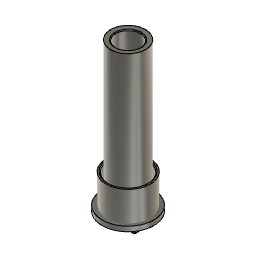
Tripod-mount v6 (Autodesk Fusion 360 design; units mm, degrees)
Autodesk Fusion 360 part; units mm, degrees
cylinder "CylinderPrimitive1" add diameter 53 height 5 placed x (1, 0, 0) y (0, 1, 0) z (0, 0, 1) at (0, 0, 0) makes body 1
hole "Hole1" at (0, 0.0929, 5) direction (0, 0, -1) diameter 40.2 depth 3 tip angle 180 countersink diameter 40.3 countersink angle 90 bodies 1
cylinder "CylinderPrimitive2" add diameter 35.8 height 150 placed x (1, 0, 0) y (0, 1, 0) z (0, 0, 1) at (0, 0.0929, 2) bodies 1
hole "Hole2" at (0.2787, -0.1858, 152) direction (0, 0, -1) diameter 25.5 depth 200 tip angle 180 countersink diameter 27 countersink angle 90 bodies 1
cylinder "CylinderPrimitive3" add diameter 2.9 height 5 placed x (1, 0, 0) y (0, 1, 0) z (0, 0, 1) at (20, -30, 0) separate body makes body 2
move_body "Move1" bodies 2 to x (1, 0, 0) y (0, 1, 0) z (0, 0, 1) at (3.3607, -17.8119, 0)
move_body "Move2" bodies 2 to x (1, 0, 0) y (0, 1, 0) z (0, 0, 1) at (-13.1273, 4.733, 0)
pattern_circular "C-Pattern1" count 3 over 360 about axis through (0, 0, 1.75) along (0, 0, 1) of bodies 2 makes body 3 at (31.404, 31.6199, 3.3333) makes body 4 at (-42.6759, 11.2491, 1.6667)
move_body "MoveFace1" bodies 3 to x (1, 0, 0) y (0, 1, 0) z (0, 0, 1) at (-14.7703, -15.636, -10.1255) on bodies 3
sketch "Sketch4" plane through (0, 0, 0) normal (1, 0, 0) x (0, 1, 0)
move_body "Move6" bodies 3 to x (1, 0, 0) y (0, 1, 0) z (0, 0, 1) at (0.1863, -0.8041, 5.3323)
move_body "Move7" bodies 3 to x (1, 0, 0) y (0, 1, 0) z (0, 0, 1) at (-17.5558, 9.3545, 0)
move_body "Move8" bodies 4 to x (1, 0, 0) y (0, 1, 0) z (0, 0, 1) at (22.6561, -23.0272, -5.0478)
move_body "Move10" bodies 2 to x (1, 0, 0) y (0, 1, 0) z (0, 0, 1) at (-7.5029, 18.5186, -9.6276)
move_body "Move11" bodies 2 to x (1, 0, 0) y (0, 1, 0) z (0, 0, 1) at (15.121, 9.8671, 0)
move_body "Move12" bodies 3 to x (1, 0, 0) y (0, 1, 0) z (0, 0, 1) at (-0.897, -0.7689, 0)
move_body "Move13" bodies 2 to x (1, 0, 0) y (0, 1, 0) z (0, 0, 1) at (-0.6407, 1.9222, 4.8344)
move_body "Move14" bodies 3 to x (1, 0, 0) y (0, 1, 0) z (0, 0, 1) at (1.0252, -0.2563, 0)
move_body "Move15" bodies 4 to x (1, 0, 0) y (0, 1, 0) z (0, 0, 1) at (0.7689, -0.5126, 0)
move_body "Move16" bodies 3 to x (1, 0, 0) y (0, 1, 0) z (0, 0, 1) at (-0.2563, -0.2563, 0)
move_body "Move17" bodies 3 to x (1, 0, 0) y (0, 1, 0) z (0, 0, 1) at (0.1281, -0.6407, 0)
move_body "Move18" bodies 4 to x (1, 0, 0) y (0, 1, 0) z (0, 0, 1) at (0.3844, 0.3844, 0)
move_body "Move19" bodies 2 to x (1, 0, 0) y (0, 1, 0) z (0, 0, 1) at (-0.5126, 0.5126, 0)
move_body "Move20" bodies 3 to x (1, 0, 0) y (0, 1, 0) z (0, 0, 1) at (0, -0.5126, 0)
move_body "Move21" bodies 4 to x (1, 0, 0) y (0, 1, 0) z (0, 0, 1) at (0.5126, 0.5126, 0)
move_body "Move22" bodies 2 to x (1, 0, 0) y (0, 1, 0) z (0, 0, 1) at (0.3844, 0.5126, 0)
move_body "Move23" bodies 2 to x (1, 0, 0) y (0, 1, 0) z (0, 0, 1) at (0.6407, 0.7689, 0)
move_body "Move24" bodies 4 to x (1, 0, 0) y (0, 1, 0) z (0, 0, 1) at (-0.7689, 0.1281, 0)
move_body "Move25" bodies 4 to x (1, 0, 0) y (0, 1, 0) z (0, 0, 1) at (0.2563, 0.2563, 0)
move_body "Move26" bodies 2 to x (1, 0, 0) y (0, 1, 0) z (0, 0, 1) at (-0.1281, -0.1281, 0)
move_body "Move27" bodies 4 to x (1, 0, 0) y (0, 1, 0) z (0, 0, 1) at (0.3844, 0, 0)
move_body "Move28" bodies 4 to x (1, 0, 0) y (0, 1, 0) z (0, 0, 1) at (-0.3844, 0, 0)
move_body "Move29" bodies 4 to x (1, 0, 0) y (0, 1, 0) z (0, 0, 1) at (0.2563, -0.1281, 0)
move_body "Move30" bodies 3 to x (1, 0, 0) y (0, 1, 0) z (0, 0, 1) at (0.3844, -0.2563, 0)
move_body "Move31" bodies 3 to x (1, 0, 0) y (0, 1, 0) z (0, 0, 1) at (0.2563, 0.2563, 0)
move_body "Move32" bodies 3 to x (1, 0, 0) y (0, 1, 0) z (0, 0, 1) at (0, -0.1281, 0)
cylinder "CylinderPrimitive4" add diameter 45 height 35 placed x (1, 0, 0) y (0, 1, 0) z (0, 0, 1) at (59, 0, 0) separate body makes body 5
hole "Hole3" at (58.8347, 0.0473, 35) direction (0, 0, -1) diameter 40.2 depth 200.89 tip angle 180 countersink diameter 42 countersink angle 90 bodies 5
move_body "Move33" bodies 5 to x (1, 0, 0) y (0, 1, 0) z (0, 0, 1) at (-58.7356, -0.0676, 0)
cylinder "CylinderPrimitive5" add diameter 9 height 2 placed x (1, 0, 0) y (0, 1, 0) z (0, 0, 1) at (35, -6, 0) separate body makes body 6
move_body "Move34" bodies 6 to x (1, 0, 0) y (0, 1, 0) z (0, 0, 1) at (-17.4019, -5.0968, -2)
cylinder "CylinderPrimitive6" add diameter 9 height 2 placed x (1, 0, 0) y (0, 1, 0) z (0, 0, 1) at (53.0398, -15.3125, 0) separate body makes body 7
cylinder "CylinderPrimitive7" add diameter 9 height 2 placed x (1, 0, 0) y (0, 1, 0) z (0, 0, 1) at (48.3354, 5.4161, 0) separate body makes body 8
move_body "Move35" bodies 7 to x (1, 0, 0) y (0, 1, 0) z (0, 0, 1) at (-52.3767, 36.1003, -2)
move_body "Move36" bodies 8 to x (1, 0, 0) y (0, 1, 0) z (0, 0, 1) at (-66.7291, -15.1351, -2.0002)
move_face "MoveFace2" by (0, 0, -0.1) 1 faces at (17.1598, -10.8954, -4.7932) on bodies 2
move_face "MoveFace3" by (0, 0, -0.1) 1 faces at (0.7014, 21.1682, -4.7932) on bodies 3
move_face "MoveFace4" to x (1, 0, 0) y (0, 1, 0) z (0, 0, 1) at (0, 0, 0.1) 1 faces at (19.0381, -11.2495, -1.4932) on bodies 2
move_face "MoveFace5" to x (1, 0, 0) y (0, 1, 0) z (0, 0, 1) at (0, 0, 0.2) 1 faces at (0.0953, 22.0752, -1.4932) on bodies 3
move_face "MoveFace6" to x (1, 0, 0) y (0, 1, 0) z (0, 0, 1) at (0, 0, 0.1) 1 faces at (19.0381, -11.2495, -1.4932) on bodies 2
move_body "Move37" bodies 2 to x (1, 0, 0) y (0, 1, 0) z (0, 0, 1) at (0, 0, 0.2)
move_face "MoveFace7" to x (1, 0, 0) y (0, 1, 0) z (0, 0, 1) at (0, 0, -0.4) 1 faces at (19.0381, -11.2495, -1.2932) on bodies 2
move_face "MoveFace8" to x (1, 0, 0) y (0, 1, 0) z (0, 0, 1) at (0, 0, -0.2) 1 faces at (19.0381, -11.2495, -1.2932) on bodies 2
move_face "MoveFace9" to x (1, 0, 0) y (0, 1, 0) z (0, 0, 1) at (0, 0, -1) 1 faces at (19.0381, -11.2495, -1.2932) on bodies 2
move_face "MoveFace10" to x (1, 0, 0) y (0, 1, 0) z (0, 0, 1) at (0, 0, -10) 1 faces at (19.0381, -11.2495, -1.2932) on bodies 2
move_face "MoveFace11" to x (1, 0, 0) y (0, 1, 0) z (0, 0, 1) at (0, 0, 5) 1 faces at (19.0381, -11.2495, -1.2932) on bodies 2
move_body "Move38" bodies 2 to x (1, 0, 0) y (0, 1, 0) z (0, 0, 1) at (0, 0, -0.3)
move_body "Move39" bodies 2 to x (1, 0, 0) y (0, 1, 0) z (0, 0, 1) at (0, 0, -0.1)
move_body "Move40" bodies 4 to x (1, 0, 0) y (0, 1, 0) z (0, 0, 1) at (0, 0, 0.048)
move_body "Move41" bodies 2 to x (1, 0, 0) y (0, 1, 0) z (0, 0, 1) at (0, 0, 0.093)
move_body "Move42" bodies 3 to x (1, 0, 0) y (0, 1, 0) z (0, 0, 1) at (0, 0, -0.107)
